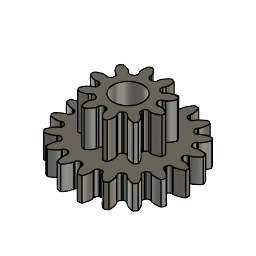
IntermediateGear2 (Autodesk Fusion 360 design; units mm, degrees)
part number: 2026-05-31-22-53-18-390
Autodesk Fusion 360 part; units mm, degrees
sketch "Base Circle" plane through (0, 0, 0) normal (0, 0, 1) x (1, 0, 0)
  circle A0 centre (0, 0) radius 1.9215
  circle A1 centre (0, 0) radius 1.25
extrude "Extrude1" add sketch "Base Circle" along normal blind 10 makes body 1
sketch "Gear Tooth" plane through (0, 0, 0) normal (0, 0, 1) x (1, 0, 0)
  spline S0 degree 5 poles (2.3146, -0.402) (2.3164, -0.4024) (2.3202, -0.403) (2.3258, -0.4036) (2.3334, -0.4042) (2.3429, -0.4044) (2.3525, -0.4042) (2.3621, -0.4039) (2.3717, -0.4033) (2.3814, -0.4027) (2.3911, -0.4021) (2.4007, -0.4013) (2.4104, -0.4003) (2.4202, -0.3992) (2.4299, -0.3979) (2.4396, -0.3964) (2.4494, -0.3947) (2.4592, -0.393) (2.469, -0.3911) (2.4788, -0.3892) (2.4886, -0.3871) (2.4984, -0.3849) (2.5082, -0.3826) (2.518, -0.3802) (2.5279, -0.3777) (2.5377, -0.3751) (2.5476, -0.3723) (2.5574, -0.3695) (2.5673, -0.3665) (2.5771, -0.3634) (2.587, -0.3603) (2.5968, -0.357) (2.6067, -0.3537) (2.6166, -0.3503) (2.6264, -0.3467) (2.6363, -0.3431) (2.6462, -0.3393) (2.656, -0.3355) (2.6659, -0.3316) (2.6757, -0.3276) (2.6856, -0.3235) (2.6954, -0.3193) (2.7053, -0.315) (2.7151, -0.3106) (2.7249, -0.3061) (2.7348, -0.3016) (2.7446, -0.2969) (2.7544, -0.2922) (2.7642, -0.2874) (2.774, -0.2825) (2.7838, -0.2775) (2.7936, -0.2724) (2.8034, -0.2673) (2.8131, -0.262) (2.8229, -0.2567) (2.8327, -0.2513) (2.8424, -0.2458) (2.8521, -0.2402) (2.8618, -0.2346) (2.8715, -0.2288) (2.8812, -0.223) (2.8909, -0.2171) (2.9006, -0.2111) (2.9102, -0.2051) (2.9199, -0.1989) (2.9295, -0.1927) (2.9391, -0.1864) (2.9487, -0.18) (2.9583, -0.1735) (2.9678, -0.167) (2.9774, -0.1604) (2.985, -0.155) (2.9907, -0.151) (2.9945, -0.1482) (2.9964, -0.1469) knots 0 0 0 0 0 0 0.01428571 0.02857143 0.04285714 0.05714286 0.07142857 0.08571429 0.1 0.11428571 0.12857143 0.14285714 0.15714286 0.17142857 0.18571429 0.2 0.21428571 0.22857143 0.24285714 0.25714286 0.27142857 0.28571429 0.3 0.31428571 0.32857143 0.34285714 0.35714286 0.37142857 0.38571429 0.4 0.41428571 0.42857143 0.44285714 0.45714286 0.47142857 0.48571429 0.5 0.51428571 0.52857143 0.54285714 0.55714286 0.57142857 0.58571429 0.6 0.61428571 0.62857143 0.64285714 0.65714286 0.67142857 0.68571429 0.7 0.71428571 0.72857143 0.74285714 0.75714286 0.77142857 0.78571429 0.8 0.81428571 0.82857143 0.84285714 0.85714286 0.87142857 0.88571429 0.9 0.91428571 0.92857143 0.94285714 0.95714286 0.97142857 0.98571429 1 1 1 1 1 1
  spline S1 degree 5 poles (2.3146, 0.402) (2.3164, 0.4024) (2.3202, 0.403) (2.3258, 0.4036) (2.3334, 0.4042) (2.3429, 0.4044) (2.3525, 0.4042) (2.3621, 0.4039) (2.3717, 0.4033) (2.3814, 0.4027) (2.3911, 0.4021) (2.4007, 0.4013) (2.4104, 0.4003) (2.4202, 0.3992) (2.4299, 0.3979) (2.4396, 0.3964) (2.4494, 0.3947) (2.4592, 0.393) (2.469, 0.3911) (2.4788, 0.3892) (2.4886, 0.3871) (2.4984, 0.3849) (2.5082, 0.3826) (2.518, 0.3802) (2.5279, 0.3777) (2.5377, 0.3751) (2.5476, 0.3723) (2.5574, 0.3695) (2.5673, 0.3665) (2.5771, 0.3634) (2.587, 0.3603) (2.5968, 0.357) (2.6067, 0.3537) (2.6166, 0.3503) (2.6264, 0.3467) (2.6363, 0.3431) (2.6462, 0.3393) (2.656, 0.3355) (2.6659, 0.3316) (2.6757, 0.3276) (2.6856, 0.3235) (2.6954, 0.3193) (2.7053, 0.315) (2.7151, 0.3106) (2.7249, 0.3061) (2.7348, 0.3016) (2.7446, 0.2969) (2.7544, 0.2922) (2.7642, 0.2874) (2.774, 0.2825) (2.7838, 0.2775) (2.7936, 0.2724) (2.8034, 0.2673) (2.8131, 0.262) (2.8229, 0.2567) (2.8327, 0.2513) (2.8424, 0.2458) (2.8521, 0.2402) (2.8618, 0.2346) (2.8715, 0.2288) (2.8812, 0.223) (2.8909, 0.2171) (2.9006, 0.2111) (2.9102, 0.2051) (2.9199, 0.1989) (2.9295, 0.1927) (2.9391, 0.1864) (2.9487, 0.18) (2.9583, 0.1735) (2.9678, 0.167) (2.9774, 0.1604) (2.985, 0.155) (2.9907, 0.151) (2.9945, 0.1482) (2.9964, 0.1469) knots 0 0 0 0 0 0 0.01428571 0.02857143 0.04285714 0.05714286 0.07142857 0.08571429 0.1 0.11428571 0.12857143 0.14285714 0.15714286 0.17142857 0.18571429 0.2 0.21428571 0.22857143 0.24285714 0.25714286 0.27142857 0.28571429 0.3 0.31428571 0.32857143 0.34285714 0.35714286 0.37142857 0.38571429 0.4 0.41428571 0.42857143 0.44285714 0.45714286 0.47142857 0.48571429 0.5 0.51428571 0.52857143 0.54285714 0.55714286 0.57142857 0.58571429 0.6 0.61428571 0.62857143 0.64285714 0.65714286 0.67142857 0.68571429 0.7 0.71428571 0.72857143 0.74285714 0.75714286 0.77142857 0.78571429 0.8 0.81428571 0.82857143 0.84285714 0.85714286 0.87142857 0.88571429 0.9 0.91428571 0.92857143 0.94285714 0.95714286 0.97142857 0.98571429 1 1 1 1 1 1
  arc A0 (2.9964, -0.1469) -> (2.9964, 0.1469) centre (0, 0) ccw
  line L0 (1.8833, -0.3271) -> (2.3146, -0.402)
  line L1 (1.8833, 0.3271) -> (2.3146, 0.402)
  line L2 (1.8833, -0.3271) -> (1.8833, 0.3271)
  point P0 (2.3614, -0.4039)
  point P1 (2.4092, -0.4004)
  point P2 (2.4574, -0.3933)
  point P3 (2.5061, -0.3831)
  point P4 (2.555, -0.3701)
  point P5 (2.6041, -0.3546)
  point P6 (2.6534, -0.3365)
  point P7 (2.7027, -0.3161)
  point P8 (2.752, -0.2934)
  point P9 (2.8012, -0.2684)
  point P10 (2.8504, -0.2412)
  point P11 (2.8993, -0.2119)
  point P12 (2.948, -0.1804)
  point P13 (2.3614, 0.4039)
  point P14 (2.4092, 0.4004)
  point P15 (2.4574, 0.3933)
  point P16 (2.5061, 0.3831)
  point P17 (2.555, 0.3701)
  point P18 (2.6041, 0.3546)
  point P19 (2.6534, 0.3365)
  point P20 (2.7027, 0.3161)
  point P21 (2.752, 0.2934)
  point P22 (2.8012, 0.2684)
  point P23 (2.8504, 0.2412)
  point P24 (2.8993, 0.2119)
  point P25 (2.948, 0.1804)
extrude "Extrude2" add sketch "Gear Tooth" along normal blind 10 bodies 1
fillet "Fillet1" radius 0.25 2 edges at (1.8932, -0.3288, 5) (1.8932, 0.3288, 5) on bodies 1
pattern_circular "C-Pattern1" count 10 over 360 about axis through (0, 0, 0) along (0, 0, 1) of "Extrude2", "Fillet1"
sketch "Diametrial Pitch Circle" plane through (0, 0, 0) normal (0, 0, 1) x (1, 0, 0)
  circle A0 centre (0, 0) radius 2.5 construction
extrude "Extrude3" cut 1 faces at (-1.717, 0, 10) along direction (0, 0, -1) blind 7 on bodies 1 bodies 1
move_body "Move1" bodies 1 to x (1, 0, 0) y (0, 1, 0) z (0, 0, 1) at (0, 0, 2)
sketch "Base Circle (1)" plane through (0, 0, 0) normal (0, 0, 1) x (1, 0, 0)
  circle A0 centre (0, 0) radius 3.9215
  circle A1 centre (0, 0) radius 1.25
extrude "Extrude4" add sketch "Base Circle (1)" along normal blind 10 separate body makes body 2
sketch "Gear Tooth (1)" plane through (0, 0, 0) normal (0, 0, 1) x (1, 0, 0)
  spline S0 degree 5 poles (4.2066, -0.4313) (4.2088, -0.4315) (4.2132, -0.4319) (4.2199, -0.4323) (4.2289, -0.4325) (4.2401, -0.4323) (4.2513, -0.4317) (4.2626, -0.431) (4.2739, -0.43) (4.2851, -0.4291) (4.2964, -0.428) (4.3077, -0.4268) (4.319, -0.4255) (4.3303, -0.424) (4.3416, -0.4224) (4.353, -0.4206) (4.3643, -0.4186) (4.3757, -0.4166) (4.387, -0.4144) (4.3983, -0.4122) (4.4097, -0.4098) (4.421, -0.4074) (4.4324, -0.4048) (4.4438, -0.4022) (4.4551, -0.3994) (4.4665, -0.3965) (4.4779, -0.3936) (4.4892, -0.3905) (4.5006, -0.3874) (4.512, -0.3841) (4.5233, -0.3808) (4.5347, -0.3774) (4.5461, -0.3739) (4.5574, -0.3703) (4.5688, -0.3666) (4.5801, -0.3629) (4.5915, -0.359) (4.6029, -0.3551) (4.6142, -0.3511) (4.6256, -0.347) (4.6369, -0.3428) (4.6483, -0.3386) (4.6596, -0.3343) (4.671, -0.3299) (4.6823, -0.3254) (4.6936, -0.3208) (4.705, -0.3162) (4.7163, -0.3115) (4.7276, -0.3067) (4.7389, -0.3018) (4.7502, -0.2969) (4.7615, -0.2919) (4.7728, -0.2868) (4.7841, -0.2817) (4.7954, -0.2764) (4.8067, -0.2711) (4.8179, -0.2658) (4.8292, -0.2603) (4.8404, -0.2548) (4.8517, -0.2492) (4.8629, -0.2436) (4.8742, -0.2378) (4.8854, -0.232) (4.8966, -0.2262) (4.9078, -0.2203) (4.919, -0.2143) (4.9302, -0.2082) (4.9414, -0.2021) (4.9525, -0.1959) (4.9637, -0.1896) (4.9748, -0.1833) (4.9837, -0.1781) (4.9904, -0.1743) (4.9949, -0.1717) (4.9971, -0.1704) knots 0 0 0 0 0 0 0.01428571 0.02857143 0.04285714 0.05714286 0.07142857 0.08571429 0.1 0.11428571 0.12857143 0.14285714 0.15714286 0.17142857 0.18571429 0.2 0.21428571 0.22857143 0.24285714 0.25714286 0.27142857 0.28571429 0.3 0.31428571 0.32857143 0.34285714 0.35714286 0.37142857 0.38571429 0.4 0.41428571 0.42857143 0.44285714 0.45714286 0.47142857 0.48571429 0.5 0.51428571 0.52857143 0.54285714 0.55714286 0.57142857 0.58571429 0.6 0.61428571 0.62857143 0.64285714 0.65714286 0.67142857 0.68571429 0.7 0.71428571 0.72857143 0.74285714 0.75714286 0.77142857 0.78571429 0.8 0.81428571 0.82857143 0.84285714 0.85714286 0.87142857 0.88571429 0.9 0.91428571 0.92857143 0.94285714 0.95714286 0.97142857 0.98571429 1 1 1 1 1 1
  spline S1 degree 5 poles (4.2066, 0.4313) (4.2088, 0.4315) (4.2132, 0.4319) (4.2199, 0.4323) (4.2289, 0.4325) (4.2401, 0.4323) (4.2513, 0.4317) (4.2626, 0.431) (4.2739, 0.43) (4.2851, 0.4291) (4.2964, 0.428) (4.3077, 0.4268) (4.319, 0.4255) (4.3303, 0.424) (4.3416, 0.4224) (4.353, 0.4206) (4.3643, 0.4186) (4.3757, 0.4166) (4.387, 0.4144) (4.3983, 0.4122) (4.4097, 0.4098) (4.421, 0.4074) (4.4324, 0.4048) (4.4438, 0.4022) (4.4551, 0.3994) (4.4665, 0.3965) (4.4779, 0.3936) (4.4892, 0.3905) (4.5006, 0.3874) (4.512, 0.3841) (4.5233, 0.3808) (4.5347, 0.3774) (4.5461, 0.3739) (4.5574, 0.3703) (4.5688, 0.3666) (4.5801, 0.3629) (4.5915, 0.359) (4.6029, 0.3551) (4.6142, 0.3511) (4.6256, 0.347) (4.6369, 0.3428) (4.6483, 0.3386) (4.6596, 0.3343) (4.671, 0.3299) (4.6823, 0.3254) (4.6936, 0.3208) (4.705, 0.3162) (4.7163, 0.3115) (4.7276, 0.3067) (4.7389, 0.3018) (4.7502, 0.2969) (4.7615, 0.2919) (4.7728, 0.2868) (4.7841, 0.2817) (4.7954, 0.2764) (4.8067, 0.2711) (4.8179, 0.2658) (4.8292, 0.2603) (4.8404, 0.2548) (4.8517, 0.2492) (4.8629, 0.2436) (4.8742, 0.2378) (4.8854, 0.232) (4.8966, 0.2262) (4.9078, 0.2203) (4.919, 0.2143) (4.9302, 0.2082) (4.9414, 0.2021) (4.9525, 0.1959) (4.9637, 0.1896) (4.9748, 0.1833) (4.9837, 0.1781) (4.9904, 0.1743) (4.9949, 0.1717) (4.9971, 0.1704) knots 0 0 0 0 0 0 0.01428571 0.02857143 0.04285714 0.05714286 0.07142857 0.08571429 0.1 0.11428571 0.12857143 0.14285714 0.15714286 0.17142857 0.18571429 0.2 0.21428571 0.22857143 0.24285714 0.25714286 0.27142857 0.28571429 0.3 0.31428571 0.32857143 0.34285714 0.35714286 0.37142857 0.38571429 0.4 0.41428571 0.42857143 0.44285714 0.45714286 0.47142857 0.48571429 0.5 0.51428571 0.52857143 0.54285714 0.55714286 0.57142857 0.58571429 0.6 0.61428571 0.62857143 0.64285714 0.65714286 0.67142857 0.68571429 0.7 0.71428571 0.72857143 0.74285714 0.75714286 0.77142857 0.78571429 0.8 0.81428571 0.82857143 0.84285714 0.85714286 0.87142857 0.88571429 0.9 0.91428571 0.92857143 0.94285714 0.95714286 0.97142857 0.98571429 1 1 1 1 1 1
  arc A0 (4.9971, -0.1704) -> (4.9971, 0.1704) centre (0, 0) ccw
  line L0 (3.8911, -0.3989) -> (4.2066, -0.4313)
  line L1 (3.8911, 0.3989) -> (4.2066, 0.4313)
  line L2 (3.8911, -0.3989) -> (3.8911, 0.3989)
  point P0 (4.262, -0.431)
  point P1 (4.3179, -0.4256)
  point P2 (4.3741, -0.4168)
  point P3 (4.4305, -0.4052)
  point P4 (4.4871, -0.3911)
  point P5 (4.5438, -0.3746)
  point P6 (4.6006, -0.3559)
  point P7 (4.6574, -0.3351)
  point P8 (4.7142, -0.3123)
  point P9 (4.7709, -0.2876)
  point P10 (4.8277, -0.261)
  point P11 (4.8843, -0.2326)
  point P12 (4.9408, -0.2024)
  point P13 (4.262, 0.431)
  point P14 (4.3179, 0.4256)
  point P15 (4.3741, 0.4168)
  point P16 (4.4305, 0.4052)
  point P17 (4.4871, 0.3911)
  point P18 (4.5438, 0.3746)
  point P19 (4.6006, 0.3559)
  point P20 (4.6574, 0.3351)
  point P21 (4.7142, 0.3123)
  point P22 (4.7709, 0.2876)
  point P23 (4.8277, 0.261)
  point P24 (4.8843, 0.2326)
  point P25 (4.9408, 0.2024)
extrude "Extrude5" add sketch "Gear Tooth (1)" along normal blind 10 bodies 2
fillet "Fillet2" radius 0.25 2 edges at (3.901, -0.4, 5) (3.901, 0.4, 5) on bodies 2
pattern_circular "C-Pattern2" count 18 over 360 about axis through (0, 0, 0) along (0, 0, 1) of "Extrude5", "Fillet2"
sketch "Diametrial Pitch Circle (1)" plane through (0, 0, 0) normal (0, 0, 1) x (1, 0, 0)
  circle A0 centre (0, 0) radius 4.5 construction
extrude "Extrude6" cut 1 faces at (3.0102, 0, 10) along direction (0, 0, -1) blind 8 on bodies 2 bodies 2
combine "Combine1" operation add target body 1 tool bodies 2
named bodies: "Spur Gear (10 teeth)", "Spur Gear (18 teeth)"
